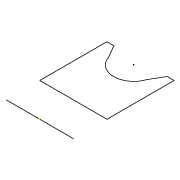
# Autodesk Inventor part: motor_trinse
Saved by Autodesk Inventor 2014 SP1 (Build 180222100, 222)
## iProperties
Created: 2015-03-04
Part Number: motor_trinse
Material: Generic
Document SubType Name: Modeling
Designer: Simen
Density: 1 g/cm^3
Appearance: Default
Author: Simen
Autodesk Inventor part; units mm, degrees
ref_plane "YZ Plane" through (0, 0, 0) normal (1, 0, 0) x (0, 1, 0)
ref_plane "XZ Plane" through (0, 0, 0) normal (0, 1, 0) x (-1, 0, 0)
ref_plane "XY Plane" through (0, 0, 0) normal (0, 0, 1) x (1, 0, 0)
sketch "Sketch1" plane through (0, 0, 0) normal (0, 0, 1) x (1, 0, 0)
  line L0 (5, 0) -> (-5, 0)
  line L1 (-4.9655, 15) -> (-4.9655, 5)
  line L2 (-4.9655, 5) -> (5.0345, 5)
  line L3 (5.0345, 5) -> (5.0345, 15)
  line L4 (5.0345, 15) -> (4.0026, 15)
  line L5 (4.0026, 15) -> (2.8501, 13.0635)
  arc A0 (-2.8501, 13.0635) -> (2.8501, 13.0635) centre (0, 14) ccw
  line L6 (-2.8501, 13.0635) -> (-3.9336, 15)
  line L7 (-3.9336, 15) -> (-4.9655, 15)
  line L8 (-4.9655, 15) -> (-9.9655, 15)
  line L9 (-9.9655, 15) -> (-9.9655, 5)
  line L10 (-9.9655, 5) -> (-4.9655, 5)
  line L11 (0, 11) -> (0, 14)
  line L12 (0, 14) -> (0, 15)
  line L13 (0, 15) -> (4.0026, 15)
  point P0 (0, 0)
  dimension "d12" = 10
  dimension "d13" = 10
  dimension "d14" = 5
  dimension "d15" = 143.621
  dimension "d16" = 3
  dimension "d17" = 1.0319
  dimension "d18" = 1.0319
  dimension "d20" = 1
  dimension "d22" = 1.9365
  dimension "d23" = 4.0026
  constraints: 28 end point, 6 parallel, 3 point on circle, 2 perpendicular, 1 centre point, 1 collinear
  measures "d12" distance of L2.end L3.end
  measures "d13" distance of L1.end L2.end
  measures "d14" distance of L1.start L8.end
  measures "d16" distance of L11.start L11.end
  measures "d17" distance of L3.end L4.end
  measures "d18" distance of L6.end L1.start
  measures "d20" distance of L11.end L12.end
  measures "d22" vertical distance of L6.start L6.end
  measures "d23" distance of L12.end L4.end
revolve "Revolution1" add sketch "Sketch1" angle 360 about axis through (5, 0, 0) along (-1, 0, 0) contours L7 L6 A0 L5 L4 L3 L2 L1 | L1 L10 L9 L8
sketch "Sketch2" plane through (5.0345, 0, 0) normal (1, 0, 0) x (0, 0, -1)
  circle A0 centre (0, 0) radius 5 projected
  circle A1 centre (0, 0) radius 8
  line L0 (-8, 0) -> (8, 0)
  dimension "d1" = 16
  constraints: 2 end point, 2 point on circle, 1 centre point, 1 coincident, 1 horizontal
  measures "d1" diameter of A1
hole "Hole1" at (5.0345, 0, 8) direction (-1, 0, 0) diameter 2 end through all
pattern_circular "Circular Pattern1" count 4 over 360 about axis through (-7.4655, 0, 0) along (1, 0, 0) of "Hole1"
body "Solid1"
